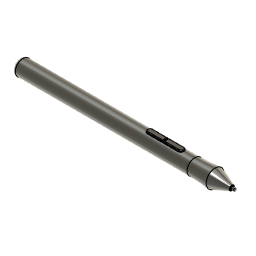
pen (Autodesk Fusion 360 design; units mm, degrees)
Autodesk Fusion 360 part; units mm, degrees
sketch "Sketch1" plane through (0, 0, 0) normal (0, 1, 0) x (1, 0, 0)
  line L0 (-138.8, 0) -> (-138.8, 3)
  arc A0 (-136.8, 5) -> (-138.8, 3) centre (-136.8, 3) ccw
  line L1 (-136.8, 5) -> (-26.5, 5)
  arc A1 (-26.5, 5) -> (-13.5, 5.75) centre (-26.5, 118.0417) ccw
  line L2 (-13.5, 5.75) -> (-2.5, 1.5)
  line L3 (-2.5, 1.5) -> (-2.5, 0.8)
  line L4 (-2.5, 0.8) -> (-0.8, 0.8)
  arc A2 (0, 0) -> (-0.8, 0.8) centre (-0.8, 0) ccw
  line L5 (0, 5) -> (0, -5) construction
  line L6 (1.75, 0) -> (22.5, 0)
  line L7 (-138.8, 0) -> (0, 0)
  dimension "d1" = 0.8
  dimension "d2" = 2.5
  dimension "d3" = 1.5
  dimension "d4" = 11
  dimension "d5" = 5.75
  dimension "d6" = 5
  dimension "d7" = 13
  dimension "d8" = 3
  dimension "d9" = 125.3
  constraint vertical L0
  constraint tangent L0 A0
  constraint tangent A0 L1
  constraint perpendicular L0 L1
  constraint tangent L1 A1
  constraint perpendicular L1 L3
  constraint perpendicular L3 L4
  constraint coincident A2.start L7.end
  constraint tangent L4 A2
  constraint vertical L5
  constraint tangent A2 L5
  constraint coincident L0.start L6
  measures "d1" radius of A2
  measures "d2" horizontal distance of A2.start L3.end
  measures "d3" vertical distance of A2.start L2.end
  measures "d4" horizontal distance of A1.end L2.end
  measures "d5" vertical distance of A2.start A1.end
  measures "d6" vertical distance of A2.start L1.end
  measures "d7" horizontal distance of L1.end A1.end
  measures "d8" distance of L0.start L0.end
  measures "d9" horizontal distance of L0.start A1.end
revolve "Revolve1" add sketch "Sketch1" angle 360 about axis through (1.75, 0, 0) along (1, 0, 0)
sketch "Sketch2" plane through (0, 0, 0) normal (0, 0, 1) x (1, 0, 0)
  line L0 (-45, 1.75) -> (-45, -1.75)
  line L1 (-45, -1.75) -> (-35.25, -1.75)
  arc A0 (-35.25, -1.75) -> (-35.25, 1.75) centre (-35.25, 0) ccw
  line L2 (-35.25, 1.75) -> (-45, 1.75)
  line L3 (-45.5, 1.75) -> (-45.5, -1.75)
  line L4 (-45.5, -1.75) -> (-55.25, -1.75)
  arc A1 (-55.25, 1.75) -> (-55.25, -1.75) centre (-55.25, 0) ccw
  line L5 (-55.25, 1.75) -> (-45.5, 1.75)
  line L6 (-57, 0) -> (-33.5, 0) construction
  point P0 (-13.5, 0)
  dimension "d11" = 0.5
  dimension "d12" = 3.5
  dimension "d13" = 23.5
  dimension "d14" = 20
  constraint vertical L0
  constraint perpendicular L0 L1
  constraint tangent L1 A0
  constraint tangent A0 L2
  constraint perpendicular L2 L3
  constraint perpendicular L3 L4
  constraint tangent L4 A1
  constraint tangent A1 L5
  constraint collinear L2 L5
  constraint collinear L1 L4
  constraint equal L2 L5
  constraint midpoint A1 L6.start
  constraint midpoint A0 L6.end
  constraint coincident origin L6
  measures "d11" distance of L0.start L3.start
  measures "d12" distance of L1.end A0.end
  measures "d13" distance of L6.start L6.end
  measures "d14" distance of L6.end P0
extrude "Extrude1" add sketch "Sketch2" along normal blind 5.75
fillet "Fillet1" radius 0.4 8 edges at (-40.125, -1.75, 5.75) (-33.5, 0, 5.75) (-40.125, 1.75, 5.75) (-50.375, 1.75, 5.75) (-57, 0, 5.75) (-50.375, -1.75, 5.75) (-45.5, 0, 5.75) (-45, 0, 5.75)
fillet "Fillet1" radius 0.4 1 edges at (-2.5, -0.5424, 1.3985)
